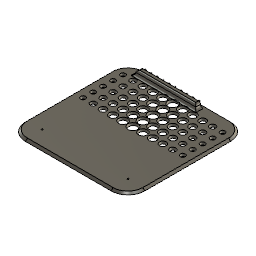
console_cover (Autodesk Fusion 360 design; units mm, degrees)
part number: 2026-01-07-20-55-40-467
Autodesk Fusion 360 part; units mm, degrees
sketch "Skizze1" plane through (0, 0, 0) normal (0, 0, 1) x (1, 0, 0)
  line L0 (17, 0) -> (103, 0)
  line L1 (120, 17) -> (120, 103)
  line L2 (103, 120) -> (17, 120)
  line L3 (0, 103) -> (0, 17)
  arc A0 (0, 17) -> (17, 0) centre (17, 17) ccw
  arc A1 (103, 0) -> (120, 17) centre (103, 17) ccw
  arc A2 (120, 103) -> (103, 120) centre (103, 103) ccw
  arc A3 (17, 120) -> (0, 103) centre (17, 103) ccw
  circle A4 centre (17, 103) radius 0.75
  circle A5 centre (103, 103) radius 0.75
  circle A6 centre (17, 17) radius 0.75
  circle A7 centre (103, 17) radius 0.75
  point P0 (120, 0)
  point P1 (0, 120)
  dimension "d1" = 120
  dimension "d2" = 120
  dimension "d3" = 17
  dimension "d4" = 17
  dimension "d5" = 1.5
  dimension "d6" = 1.5
  dimension "d7" = 1.5
  dimension "d8" = 1.5
  constraint horizontal L0
  constraint vertical L1
  constraint horizontal L2
  constraint vertical L3
  constraint coincident origin L0
  constraint coincident origin L3
  constraint tangent L0 A0
  constraint tangent L3 A0
  constraint coincident P0 L0
  constraint coincident P0 L1
  constraint tangent L0 A1
  constraint tangent L1 A1
  constraint tangent L1 A2
  constraint tangent L2 A2
  constraint equal A1 A2
  constraint coincident P1 L2
  constraint coincident P1 L3
  constraint tangent L2 A3
  constraint tangent L3 A3
  constraint equal A1 A3
  constraint concentric A3 A4
  constraint concentric A2 A5
  constraint concentric A0 A6
  constraint concentric A1 A7
  measures "d1" distance of origin P0
  measures "d2" distance of origin P1
  measures "d3" radius of A0
  measures "d4" radius of A1
  measures "d5" diameter of A4
  measures "d6" diameter of A5
  measures "d7" diameter of A6
  measures "d8" diameter of A7
extrude "Extrusion1" add sketch "Skizze1" along normal blind 2 draft -45 contours L0 L1 L2 L3 A0 A1 A2 A3 | A4 | A5 | A6 | A7
hole "Bohrung1" at (17, 17, 0) direction (0, 0, 1) diameter 1.5 depth 2 tip angle 180 countersink diameter 3 countersink angle 90
hole "Bohrung2" at (103, 17, 0) direction (0, 0, 1) diameter 1.5 depth 2 tip angle 180 countersink diameter 3 countersink angle 90
sketch "Skizze3" plane through (0, 0, 2) normal (0, 0, 1) x (-1, 0, 0)
  circle A0 centre (-103, -17) radius 0.75
  circle A1 centre (-17, -17) radius 0.75
  line L0 (-103, -118) -> (-17, -118)
  arc A2 (-17, -118) -> (-2, -103) centre (-17, -103) ccw
  line L1 (-2, -103) -> (-2, -17)
  arc A3 (-2, -17) -> (-17, -2) centre (-17, -17) ccw
  line L2 (-17, -2) -> (-103, -2)
  arc A4 (-103, -2) -> (-118, -17) centre (-103, -17) ccw
  line L3 (-118, -17) -> (-118, -103)
  arc A5 (-118, -103) -> (-103, -118) centre (-103, -103) ccw
  line L4 (-17, -118) -> (-17, -116)
  line L5 (-17, -116) -> (-20, -116)
  line L6 (-17, -116) -> (-77, -116)
  line L7 (-77, -116) -> (-77, -111)
  line L8 (-77, -111) -> (-17, -111)
  line L9 (-17, -111) -> (-17, -116)
  dimension "d31" = 2
  dimension "d32" = 60
  dimension "d33" = 5
  constraint coincident L0.end A2.start
  constraint perpendicular L0 L4
  constraint perpendicular L4 L5
  constraint horizontal L6
  constraint vertical L7
  constraint horizontal L8
  constraint vertical L9
  measures "d31" distance of L0.end L4.end
  measures "d32" distance of L4.end L6.end
  measures "d33" distance of L4.end L8.end
extrude "Extrusion2" add sketch "Skizze3" along normal blind 4.5 contours L5 L6 L7 L8 L9
sketch "Skizze4" plane through (0, 116, 0) normal (0, 1, 0) x (-1, 0, 0)
  line L0 (-77, 2) -> (-17, 2)
  line L1 (-17, 2) -> (-17, 6.5)
  line L2 (-17, 6.5) -> (-77, 6.5)
  line L3 (-77, 6.5) -> (-77, 2)
  line L4 (-17, 2) -> (-20, 2)
  line L5 (-20, 2) -> (-20, 5)
  line L6 (-20, 5) -> (-17, 5)
  line L7 (-17, 5) -> (-17, 2)
  circle A0 centre (-20, 5) radius 1.25
  circle A1 centre (-26, 5) radius 1.25
  circle A2 centre (-32, 5) radius 1.25
  circle A3 centre (-38, 5) radius 1.25
  circle A4 centre (-44, 5) radius 1.25
  circle A5 centre (-50, 5) radius 1.25
  circle A6 centre (-56, 5) radius 1.25
  circle A7 centre (-62, 5) radius 1.25
  circle A8 centre (-68, 5) radius 1.25
  circle A9 centre (-74, 5) radius 1.25
  dimension "d36" = 3
  dimension "d37" = 3
  dimension "d38" = 2.5
  dimension "d41" = -6
  dimension "d42" = 0
  constraint horizontal L4
  constraint vertical L5
  constraint horizontal L6
  constraint vertical L7
  constraint coincident L0.end L1.start
  constraint coincident L5.end L6.start
  measures "d36" distance of L0.end L4.end
  measures "d37" distance of L0.end L6.end
  measures "d38" diameter of A0
extrude "Extrusion3" add sketch "Skizze4" along normal blind 1.5 draft -15 contours L5 L6 A0 | L5 L6 A0 | A1 | A2 | A3 | A4 | A5 | A6 | A7 | A8 | A9
fillet "Abrundung1" radius 2 3 edges at (17, 113.5, 6.5) (47, 111, 6.5) (77, 113.5, 6.5)
fillet "Abrundung2" radius 2.5 3 edges at (17, 113.5, 2) (47, 111, 2) (77, 113.5, 2)
fillet "Abrundung3" radius 0.2 5 edges at (77.7322, 116, 2.7322) (76.4142, 116, 5.9142) (47, 116, 6.5) (17.5858, 116, 5.9142) (16.2678, 116, 2.7322)
sketch "Skizze5" plane through (0, 0, 0) normal (0, 0, -1) x (1, 0, 0)
  circle A0 centre (103, -17) radius 1.5
  circle A1 centre (17, -17) radius 1.5
  arc A2 (0, -103) -> (17, -120) centre (17, -103) ccw
  line L0 (17, -120) -> (103, -120)
  arc A3 (103, -120) -> (120, -103) centre (103, -103) ccw
  line L1 (120, -103) -> (120, -17)
  arc A4 (120, -17) -> (103, 0) centre (103, -17) ccw
  line L2 (103, 0) -> (17, 0)
  arc A5 (17, 0) -> (0, -17) centre (17, -17) ccw
  line L3 (0, -17) -> (0, -103)
  line L4 (103, -120) -> (60, -120)
  line L5 (60, -120) -> (60, -85)
  line L6 (60, -85) -> (103, -85)
  line L7 (103, -85) -> (103, -120)
  circle A6 centre (60, -85) radius 4
  circle A7 centre (70, -85) radius 3.5
  circle A8 centre (80, -85) radius 3
  circle A9 centre (90, -85) radius 2.5
  circle A10 centre (100, -85) radius 2
  circle A11 centre (110, -85) radius 1.5
  circle A12 centre (50, -85) radius 3.5
  circle A13 centre (40, -85) radius 3
  circle A14 centre (30, -85) radius 2.5
  circle A15 centre (20, -85) radius 2
  circle A16 centre (10, -85) radius 1.5
  circle A17 centre (110, -105) radius 1.5
  circle A18 centre (100, -105) radius 2
  circle A19 centre (90, -105) radius 2.5
  circle A20 centre (80, -105) radius 3
  circle A21 centre (70, -105) radius 3.5
  circle A22 centre (60, -105) radius 4
  circle A23 centre (50, -105) radius 3.5
  circle A24 centre (40, -105) radius 3
  circle A25 centre (30, -105) radius 2.5
  circle A26 centre (20, -105) radius 2
  circle A27 centre (10, -105) radius 1.5
  circle A28 centre (110, -95) radius 1.5
  circle A29 centre (100, -95) radius 2
  circle A30 centre (90, -95) radius 2.5
  circle A31 centre (80, -95) radius 3
  circle A32 centre (70, -95) radius 3.5
  circle A33 centre (60, -95) radius 4
  circle A34 centre (50, -95) radius 3.5
  circle A35 centre (40, -95) radius 3
  circle A36 centre (30, -95) radius 2.5
  circle A37 centre (20, -95) radius 2
  circle A38 centre (10, -95) radius 1.5
  circle A39 centre (110, -75) radius 1.5
  circle A40 centre (100, -75) radius 2
  circle A41 centre (90, -75) radius 2.5
  circle A42 centre (80, -75) radius 3
  circle A43 centre (70, -75) radius 3.5
  circle A44 centre (60, -75) radius 4
  circle A45 centre (50, -75) radius 3.5
  circle A46 centre (40, -75) radius 3
  circle A47 centre (30, -75) radius 2.5
  circle A48 centre (20, -75) radius 2
  circle A49 centre (10, -75) radius 1.5
  circle A50 centre (110, -65) radius 1.5
  circle A51 centre (100, -65) radius 2
  circle A52 centre (90, -65) radius 2.5
  circle A53 centre (80, -65) radius 3
  circle A54 centre (70, -65) radius 3.5
  circle A55 centre (60, -65) radius 4
  circle A56 centre (50, -65) radius 3.5
  circle A57 centre (40, -65) radius 3
  circle A58 centre (30, -65) radius 2.5
  circle A59 centre (20, -65) radius 2
  circle A60 centre (10, -65) radius 1.5
  dimension "d51" = 43
  dimension "d52" = 35
  dimension "d57" = 7
  dimension "d58" = 6
  dimension "d59" = 5
  dimension "d60" = 3
  dimension "d61" = 7
  dimension "d62" = 5
  dimension "d63" = 4
  dimension "d64" = 3
  dimension "d67" = 0
  dimension "d68" = 10
  constraint horizontal L4
  constraint vertical L5
  constraint horizontal L6
  constraint vertical L7
  constraint coincident L0.end A3.start
  constraint coincident L5.end L6.start
  measures "d51" distance of L0.end L4.end
  measures "d52" distance of L0.end L6.end
  measures "d57" diameter of A7
  measures "d58" diameter of A8
  measures "d59" diameter of A9
  measures "d60" diameter of A11
  measures "d61" diameter of A12
  measures "d62" diameter of A14
  measures "d63" diameter of A15
  measures "d64" diameter of A16
extrude "Extrusion4" cut sketch "Skizze5" against normal blind 2 draft 25 contours L5 A22 | L5 A22 | L6 A10 | L6 A10 | L5 A33 | L5 A33 | L6 A9 | L6 A9 | L5 L6 A6 | L5 L6 A6 | L6 A8 | L6 A8 | L6 A7 | L6 A7 | A11 | A12 | A13 | A14 | A15 | A16 | A17 | A18 | A19 | A20 | A21 | A23 | A24 | A25 | A26 | A27 | A28 | A29 | A30 | A31 | A32 | A34 | A35 | A36 | A37 | A38 | A39 | A40 | A41 | A42 | A43 | A44 | A45 | A46 | A47 | A48 | A49 | A50 | A51 | A52 | A53 | A54 | A55 | A56 | A57 | A58 | A59 | A60
fillet "Abrundung4" radius 1 2 edges at (18.3985, 17.5424, 0) (104.3985, 17.5424, 0)
hole "Bohrung3" [suppressed]
hole "Bohrung4" [suppressed]
